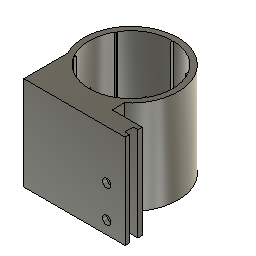
Fijador_motor (Autodesk Fusion 360 design; units mm, degrees)
Autodesk Fusion 360 part; units mm, degrees
sketch "Boceto1" plane through (0, 0, 0) normal (0, 0, 1) x (1, 0, 0)
  circle A0 centre (0, 0) radius 19.5 construction
  line L0 (0, 0) -> (0, 18.75) construction
  line L1 (0, 18.75) -> (0.4305, 19.4952)
  line L2 (0, 18.75) -> (0.8606, 18.75) construction
  line L3 (0, 18.75) -> (-0.4305, 19.4952)
  line L4 (0, 18.75) -> (0.8606, 18.75) construction
  line L5 (-16.238, 9.375) -> (-17.0986, 9.3748)
  line L6 (-16.238, 9.375) -> (-16.6681, 10.1204)
  line L7 (-16.238, -9.375) -> (-16.6681, -10.1204)
  line L8 (-16.238, -9.375) -> (-17.0986, -9.3748)
  line L9 (0, -18.75) -> (0.4305, -19.4952)
  line L10 (0, -18.75) -> (-0.4305, -19.4952)
  line L11 (16.238, -9.375) -> (17.0986, -9.3748)
  line L12 (16.238, -9.375) -> (16.6681, -10.1204)
  line L13 (16.238, 9.375) -> (16.6681, 10.1204)
  line L14 (16.238, 9.375) -> (17.0986, 9.3748)
  circle A1 centre (0, 0) radius 19.5
  line L15 (0, 0) -> (0, -24.75) construction
  line L16 (0, 0) -> (0, -19.5) construction
  line L17 (0, 0) -> (19.5, 0) construction
  line L18 (0, -24.75) -> (-36.4194, -24.75) construction
  line L19 (-36.4194, -24.75) -> (0, -24.75) construction
  line L20 (30.7797, -24.75) -> (0, -24.75) construction
  line L21 (0, 0) -> (-19.5, 0) construction
  line L22 (-19.5, 0) -> (-19.5, -28.8)
  line L23 (0, 0) -> (19.396, 0) construction
  line L24 (19.396, 0) -> (19.396, -26.75) construction
  line L25 (19.396, -26.75) -> (21.396, -26.75) construction
  line L26 (19.396, -26.75) -> (17.396, -26.75) construction
  line L27 (13.9548, -13.6203) -> (13.9548, -24.75)
  arc A2 (13.926, -17.0313) -> (-19.4752, -10.2331) centre (0, 0) ccw
  line L28 (-19.5, -28.8) -> (-19.5, -30.8)
  line L29 (-19.5, -30.8) -> (28, -30.8)
  line L30 (13.9548, -24.75) -> (13.9548, -22.75)
  line L31 (13.9548, -22.75) -> (28, -22.75)
  line L32 (28, -22.75) -> (28, -30.8)
  line L33 (17.396, -26.75) -> (-6, -26.75) construction
  line L34 (0, 0) -> (0, -26.75) construction
  dimension "d1" = 39
  dimension "d2" = 18.75
  dimension "d3" = 59.988
  dimension "d4" = 0.8606
  dimension "d5" = 120.012
  dimension "d6" = 0.8606
  dimension "d8" = 360
  dimension "d9" = 39
  dimension "d10" = 24.75
  dimension "d13" = 19.5
  dimension "d14" = 28.8
  dimension "d15" = 19.396
  dimension "d16" = 26.75
  dimension "d17" = 2
  dimension "d18" = 2
  dimension "d19" = 11.1297
  dimension "d20" = 22
  dimension "d21" = 2
  dimension "d22" = 2
  constraint coincident A0.centre L0.start
  constraint vertical L0
  constraint horizontal L2
  constraint coincident A0 L1.end
  constraint horizontal L4
  constraint vertical L15
  constraint coincident L15 L16.end
  constraint coincident A1 L16.end
  constraint coincident A0 L17.end
  constraint perpendicular L0 L17
  constraint perpendicular L15 L18
  constraint perpendicular L15 L20
  constraint horizontal L21
  constraint perpendicular L18 L22
  constraint perpendicular L20 L24
  constraint perpendicular L24 L25
  constraint perpendicular L24 L26
  constraint vertical L27
  constraint coincident A0 L27.start
  constraint coincident L20 L27.end
  constraint perpendicular L19 L28
  constraint perpendicular L22 L29
  constraint coincident L27 L30.end
  constraint perpendicular L30 L31
  constraint perpendicular L29 L32
  constraint parallel L26 L33
  constraint coincident L33 L34.end
  constraint perpendicular L33 L34
  measures "d1" diameter of A0
  measures "d2" distance of A0.centre L0.end
  measures "d3" angle of L1 L2
  measures "d4" distance of L0.end L1.end
  measures "d5" angle of L3 L4
  measures "d6" distance of L0.end L3.end
  measures "d9" diameter of A1
  measures "d10" distance of A0.centre L15.end
  measures "d13" distance of A0.centre L21.end
  measures "d14" distance of L21.end L22.end
  measures "d15" distance of A0.centre L23.end
  measures "d16" distance of L23.end L24.end
  measures "d17" distance of L24.end L25.end
  measures "d18" distance of L24.end L26.end
  measures "d19" distance of L27.start L27.end
  measures "d20" radius of A2
  measures "d21" distance of L22.end L28.end
  measures "d22" distance of L27.end L30.end
extrude "Extruir1" add sketch "Boceto1" along normal blind 44 contours L1 L3 A1 | A1 L22 L27 A2 | L13 L14 A1 | L5 L6 A1 | A1 L22 L27 L28 L29 L31 L32 | L11 L12 A1 | L7 L8 A1 | L9 L10 A1 makes body 1
sketch "Boceto2" plane through (0, -22.75, 0) normal (0, 1, 0) x (-1, 0, 0)
  line L0 (-28, 0) -> (-13.9548, 0)
  line L1 (-13.9548, 44) -> (-28, 44)
  line L2 (0, 0) -> (0, 21) construction
  line L3 (0, 21) -> (-19.396, 21) construction
  circle A0 centre (-19.396, 21) radius 2
  line L4 (-19.396, 21) -> (-19.396, 6) construction
  circle A1 centre (-19.396, 6) radius 2
  line L5 (-19.396, 6) -> (2.854, 6) construction
  line L6 (-19.396, 6) -> (-19.396, 0) construction
  line L7 (-19.396, 0) -> (5.604, 0) construction
  line L8 (-19.396, 6) -> (-19.396, 37.747) construction
  arc A2 (5.604, 0) -> (-29.313, 46.9893) centre (-109.7168, -49.2252) ccw
  line L9 (-109.7168, -49.2252) -> (5.604, 0) construction
  line L10 (-109.7168, -49.2252) -> (-29.313, 46.9893) construction
  line L11 (-29.313, 46.9893) -> (-29.313, 0)
  line L12 (-29.313, 0) -> (5.604, 0)
  dimension "d25" = 21
  dimension "d26" = 19.396
  dimension "d27" = 4
  dimension "d28" = 15
  dimension "d29" = 4
  dimension "d36" = 22.25
  dimension "d37" = 25
  dimension "d38" = 31.747
  dimension "d39" = 27
  constraint coincident L2.start origin
  constraint vertical L2
  constraint perpendicular L2 L3
  constraint coincident L3.end A0.centre
  constraint perpendicular L3 L4
  constraint coincident L4.end A1.centre
  constraint perpendicular L4 L5
  constraint coincident L0 L6.end
  constraint perpendicular L0 L6
  constraint perpendicular L2 L7
  constraint parallel L4 L8
  constraint perpendicular L0 L11
  constraint perpendicular L11 L12
  measures "d25" distance of L2.start L2.end
  measures "d26" distance of L2.end L3.end
  measures "d27" diameter of A0
  measures "d28" distance of L3.end L4.end
  measures "d29" diameter of A1
  measures "d36" distance of L4.end L5.end
  measures "d37" distance of L6.end L7.end
  measures "d38" distance of L4.end L8.end
  measures "d39" angle of L9 L10
extrude "Extruir2" cut sketch "Boceto2" against normal blind 8.05 contours A0 | A1 bodies 1
ref_plane "PlanoDeObra1" through (0, -26.75, 0) normal (0, 1, 0) x (0, 0, 1)
sketch "Boceto3" plane through (0, -26.75, 0) normal (0, 1, 0) x (1, 0, 0)
  line L0 (0, 0) -> (19.792, 0) construction
  line L1 (19.792, 0) -> (-5.208, 0) construction
  dimension "d33" = 19.792
  dimension "d34" = 25
  constraint coincident L0.start origin
  constraint horizontal L0
  constraint parallel L0 L1
  measures "d33" distance of L0.start L0.end
  measures "d34" distance of L0.end L1.end
extrude "Extruir3" add sketch "Boceto2" against normal blind 4 separate body makes body 2
move_body "Desplazar1" bodies 2 to x (1, 0, 0) y (0, 1, 0) z (0, 0, 1) at (0, -2, 0)
combine "Combinar1" operation cut target body 1 tool bodies 2
